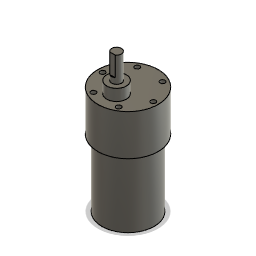
gmotorF1 (Autodesk Fusion 360 design; units mm, degrees)
Autodesk Fusion 360 part; units mm, degrees
sketch "Sketch1" plane through (0, 0, 0) normal (0, 1, 0) x (1, 0, 0)
  circle A0 centre (0, 0) radius 18.5
  dimension "d1" = 37
  constraint coincident A0.centre origin
  measures "d1" diameter of A0
extrude "Extrude1" add sketch "Sketch1" against normal blind 25
sketch "Sketch2" plane through (0, -25, 0) normal (0, -1, 0) x (1, 0, 0)
  circle A0 centre (0, 0) radius 18.5
  circle A1 centre (0, 0) radius 16
  dimension "d4" = 32
  constraint coincident A0.centre A1.centre
  measures "d4" diameter of A1
extrude "Extrude2" add sketch "Sketch2" along normal blind 41 contours A1
sketch "Sketch3" plane through (0, 0, 0) normal (0, 1, 0) x (-1, 0, 0)
  circle A0 centre (0, 0) radius 18.5
  line L0 (0, 0) -> (0, 7)
  circle A1 centre (0, 7) radius 6
  dimension "d7" = 7
  dimension "d8" = 12
  constraint coincident A0.centre L0.start
  constraint vertical L0
  constraint coincident L0.end A1.centre
  measures "d7" distance of A0.centre L0.end
  measures "d8" diameter of A1
extrude "Extrude3" add sketch "Sketch3" along normal blind 7 contours A1
sketch "Sketch4" plane through (0, 7, 0) normal (0, 1, 0) x (-1, 0, 0)
  circle A0 centre (0, 7) radius 6
  circle A1 centre (0, 7) radius 3
  dimension "d11" = 6
  constraint concentric A0 A1
  measures "d11" diameter of A1
extrude "Extrude4" add sketch "Sketch4" along normal blind 15.5 contours A1
sketch "Sketch5" plane through (0, 0, 0) normal (0, 1, 0) x (-1, 0, 0)
  circle A0 centre (0, 7) radius 6
  circle A1 centre (0, 0) radius 18.5
  line L0 (0, 0) -> (15.5, 0)
  circle A2 centre (15.5, 0) radius 1.5
  circle A3 centre (7.75, 13.4234) radius 1.5
  circle A4 centre (-7.75, 13.4234) radius 1.5
  circle A5 centre (-15.5, 0) radius 1.5
  circle A6 centre (-7.75, -13.4234) radius 1.5
  circle A7 centre (7.75, -13.4234) radius 1.5
  dimension "d14" = 3
  dimension "d15" = 15.5
  dimension "d17" = 360
  constraint coincident A1.centre L0.start
  constraint horizontal L0
  constraint coincident L0.end A2.centre
  measures "d14" diameter of A2
  measures "d15" distance of A1.centre L0.end
extrude "Extrude5" cut sketch "Sketch5" against normal blind 3.5 contours A2 | A3 | A4 | A5 | A6 | A7
sketch "Sketch6" plane through (0, 22.5, 0) normal (0, 1, 0) x (-1, 0, 0)
  circle A0 centre (0, 7) radius 3
  circle A1 centre (0, 7) radius 3
  line L0 (0, 7) -> (0, 9.5)
  line L1 (0, 9.5) -> (-1.6583, 9.5)
  line L2 (0, 9.5) -> (1.6583, 9.5)
  constraint concentric A0 A1
  constraint coincident A0.centre A1.centre
  constraint vertical L0
  constraint coincident A1 L1.end
  constraint perpendicular L0 L1
  constraint coincident A1 L2.end
  constraint perpendicular L0 L2
extrude "Extrude6" cut sketch "Sketch6" against normal blind 12 contours A0 A1 L1 L2 picked at (-0.1459, 9.8226)
